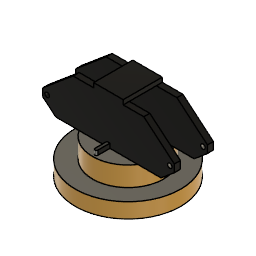
robotic_arm_jaw_mount (Autodesk Fusion 360 design; units mm, degrees)
part number: 2026-05-08-18-07-45-886
Autodesk Fusion 360 part; units mm, degrees
sketch "Sketch1" plane through (0, 0, 0) normal (0, 0, 1) x (1, 0, 0)
  circle A0 centre (0, 0) radius 35
  dimension "d1" = 70
  constraint coincident A0.centre origin
  measures "d1" diameter of A0
extrude "Extrude1" add sketch "Sketch1" along normal blind 10
sketch "Sketch2" plane through (0, 0, 10) normal (0, 0, 1) x (-1, 0, 0)
  circle A0 centre (0, 0) radius 35
  circle A1 centre (0, 0) radius 23.5
  dimension "d4" = 47
  constraint coincident A0.centre A1.centre
  measures "d4" diameter of A1
extrude "Extrude2" add sketch "Sketch2" along normal blind 13 contours A1
ref_plane "WorkPlane1" through (0, 13, 0) normal (0, 1, 0) x (0, 0, 1)
sketch "Sketch3" plane through (0, 13, 0) normal (0, 1, 0) x (1, 0, 0)
sketch "Sketch4" plane through (0, 13, 0) normal (0, 1, 0) x (1, 0, 0)
  line L0 (0, -23) -> (35, -23)
  line L1 (35, -23) -> (45, -23)
  line L2 (35, -23) -> (43.8095, -30.3921)
  line L3 (43.8095, -30.3921) -> (43.8095, -35.3921)
  line L4 (0, -23) -> (0, -56.4386)
  line L5 (23.5, -23) -> (23.5, -67.1153)
  line L6 (43.8095, -35.3921) -> (23.5, -52.4338)
  line L7 (43.8095, -35.3921) -> (43.8095, -48.4067)
  line L8 (23.5, -52.4338) -> (0, -52.4338)
  line L9 (0, -23) -> (-35, -23)
  line L10 (-35, -23) -> (-43.8095, -30.3921)
  line L11 (-43.8095, -30.3921) -> (-43.8095, -35.3921)
  line L12 (-43.8095, -35.3921) -> (-23.5, -52.4338)
  line L13 (-23.5, -52.4338) -> (0, -52.4338)
  point P0 (23.5, -23)
  dimension "d8" = 35
  dimension "d9" = 11.5
  dimension "d10" = 10
  dimension "d11" = 11.5
  dimension "d12" = 40
  dimension "d13" = 5
  dimension "d14" = 50
  constraint horizontal L0
  constraint parallel L0 L1
  constraint perpendicular L1 L3
  constraint perpendicular L0 L4
  constraint coincident P0 L5.start
  constraint perpendicular L0 L5
  constraint coincident L5 L6.end
  constraint parallel L3 L7
  constraint coincident L4 L8.end
  constraint perpendicular L4 L8
  constraint symmetric L0.start L4 L9.start
  constraint symmetric L0.end L4 L9.end
  constraint symmetric L2.end L4 L10.end
  constraint symmetric L3.end L4 L11.end
  constraint symmetric L4 L6.end L12.end
  constraint symmetric L4 L8.end L13.end
  measures "d8" distance of L0.start L0.end
  measures "d9" distance of L0.end P0
  measures "d10" distance of L0.end L1.end
  measures "d11" distance of L0.end L2.end
  measures "d12" angle of L1 L2
  measures "d13" distance of L2.end L3.end
  measures "d14" angle of L6 L7
extrude "Extrude3" add sketch "Sketch4" against normal blind 4
sketch "Sketch5" plane through (0, 13, 0) normal (0, 1, 0) x (-1, 0, 0)
  line L0 (-35, 23) -> (-19.5768, 23)
  line L1 (-19.5768, 23) -> (19.5768, 23)
  line L2 (19.5768, 23) -> (35, 23)
  line L3 (35, 23) -> (43.8095, 30.3921)
  line L4 (43.8095, 30.3921) -> (43.8095, 35.3921)
  line L5 (43.8095, 35.3921) -> (23.5, 52.4338)
  line L6 (23.5, 52.4338) -> (-23.5, 52.4338)
  line L7 (-23.5, 52.4338) -> (-43.8095, 35.3921)
  line L8 (-43.8095, 35.3921) -> (-43.8095, 30.3921)
  line L9 (-43.8095, 30.3921) -> (-35, 23)
  line L10 (43.8095, 32.8921) -> (40.8095, 32.8921)
  circle A0 centre (40.8095, 32.8921) radius 1.5
  dimension "d17" = 3
  dimension "d18" = 3
  constraint midpoint L4 L10.start
  constraint perpendicular L4 L10
  constraint coincident L10.end A0.centre
  measures "d17" distance of L10.start L10.end
  measures "d18" diameter of A0
extrude "Extrude4" cut sketch "Sketch5" against normal blind 6 contours A0
mirror "Mirror1" about plane through (0, 0, 0) normal (1, 0, 0) of "Extrude4"
mirror "Mirror2" about plane through (0, 0, 0) normal (0, 1, 0) of "Extrude3", "Extrude4", "Mirror1"
sketch "Sketch6" plane through (0, 0, 23) normal (0, 0, 1) x (-1, 0, 0)
  line L0 (19.5768, -13) -> (-19.5768, -13)
  arc A0 (-19.5768, -13) -> (19.5768, -13) centre (0, 0) ccw
  line L1 (0, -13) -> (0, -23.5)
  line L2 (0, -13) -> (1, -13)
  line L3 (1, -13) -> (1, -22)
  line L4 (1, -22) -> (0, -22)
  line L5 (-1, -22) -> (0, -22)
  line L6 (-1, -13) -> (-1, -22)
  dimension "d25" = 1
  dimension "d26" = 9
  constraint midpoint L0 L1.start
  constraint midpoint A0 L1.end
  constraint perpendicular L1 L2
  constraint perpendicular L0 L3
  constraint coincident L1 L4.end
  constraint perpendicular L1 L4
  constraint symmetric L1 L2.end L6.start
  constraint symmetric L1 L3.end L5.start
  constraint symmetric L1 L4.end L5.end
  measures "d25" distance of L1.start L2.end
  measures "d26" distance of L2.end L3.end
extrude "Extrude5" add sketch "Sketch6" along normal blind 3 contours L0 L1 L2 L3 L4 | L0 L1 L5 L6
sketch "Sketch7" plane through (0, 0, 23) normal (0, 0, 1) x (-1, 0, 0)
  line L0 (1, -13) -> (1, -22)
  line L1 (1, -22) -> (-1, -22)
  line L2 (-1, -22) -> (-1, -13)
  line L3 (-1, -13) -> (-19.5768, -13)
  arc A0 (-19.5768, -13) -> (19.5768, -13) centre (0, 0) ccw
  line L4 (19.5768, -13) -> (1, -13)
fillet "Fillet1" radius 1 2 edges at (-1, 22, 24.5) (1, 22, 24.5)
mirror "Mirror3" about plane through (0, 0, 0) normal (0, 1, 0) of "Extrude5", "Fillet1"
sketch "Sketch8" plane through (0, 0, 52.4338) normal (0, 0, 1) x (-1, 0, 0)
  line L0 (-23.5, -13) -> (23.5, -13)
  line L1 (23.5, -13) -> (23.5, -9)
  line L2 (23.5, -9) -> (-23.5, -9)
  line L3 (-23.5, -9) -> (-23.5, -13)
  line L4 (9.827, -13) -> (-9.827, -13)
  line L5 (-9.827, -13) -> (-9.827, 13)
  line L6 (-9.827, 13) -> (9.827, 13)
  line L7 (9.827, 13) -> (9.827, -13)
  line L8 (9.827, -13) -> (-9.827, 13) construction
  line L9 (-9.827, -13) -> (9.827, 13) construction
  constraint horizontal L4
  constraint perpendicular L4 L5
  constraint parallel L4 L6
  constraint parallel L5 L7
  constraint coincident L8 origin
  constraint coincident L9 origin
  constraint coincident L0 L4.start
extrude "Extrude6" add sketch "Sketch8" along normal blind 3 contours L0 L2 L4 L5 L7 | L2 L5 L6 L7
sketch "Sketch9" plane through (0, 0, 0) normal (0, 0, -1) x (1, 0, 0)
  circle A0 centre (0, 0) radius 35
  circle A1 centre (0, 0) radius 10
  dimension "d35" = 20
  constraint coincident A0.centre A1.centre
  measures "d35" diameter of A1
extrude "Extrude7" cut sketch "Sketch9" against normal blind 10 contours A1
